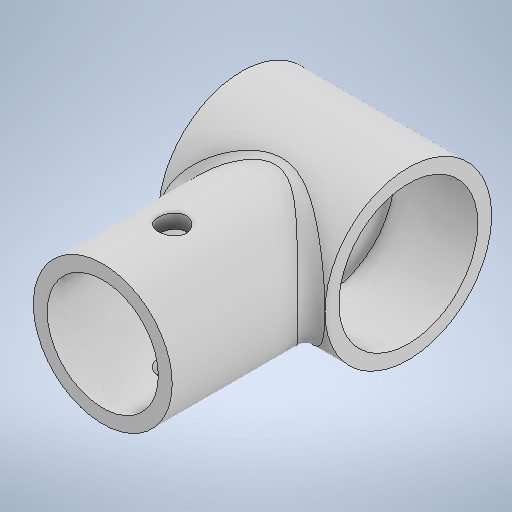
# Autodesk Inventor part: bielle rocker
Saved by Autodesk Inventor 2026.2 (Build 302298010, 298A)
## iProperties
Created: 2026-03-19
Part Number: bielle rocker
Material: Générique
Document SubType Name: Modeling
Designer: genon
Density: 1 g/cm^3
Appearance: Par défaut
Author: genon
Autodesk Inventor part; units mm, degrees
ref_plane "YZ Plane" through (0, 0, 0) normal (1, 0, 0) x (0, 1, 0)
ref_plane "XY Plane" through (0, 0, 0) normal (0, 0, 1) x (1, 0, 0)
sketch "Esquisse2" plane through (0, 0, 0) normal (0, 0, 1) x (1, 0, 0)
  circle A0 centre (0, 0) radius 4
  circle A1 centre (0, 0) radius 5
  dimension "d0" = 8
  dimension "d1" = 10
  constraints: 2 centre point, 2 coincident
  measures "d0" diameter of A0
  measures "d1" diameter of A1
extrude "Extrusion1" add sketch "Esquisse2" along normal blind 10
sketch "Esquisse3" plane through (0, 0, 0) normal (1, 0, 0) x (0, 1, 0)
  line L0 (0, 0) -> (0, -6)
  circle A0 centre (0, -6) radius 5
  circle A1 centre (0, -6) radius 6
  dimension "d4" = 6
  dimension "d5" = 10
  dimension "d6" = 12
  constraints: 2 centre point, 2 coincident, 2 end point, 1 vertical
  measures "d4" distance of L0.start L0.end
  measures "d5" diameter of A0
  measures "d6" diameter of A1
extrude "Extrusion2" add sketch "Esquisse3" along normal mid plane 12
sketch "Esquisse4" plane through (0, 0, 0) normal (1, 0, 0) x (0, 1, 0)
  circle A0 centre (0, -6) radius 5 projected
  line L0 (0, -11) -> (0, -1)
  circle A1 centre (0, -6) radius 2.75
  circle A2 centre (0, -6) radius 5
  line L1 (5, 0) -> (0, 0) projected
  line L2 (5, 0) -> (-5, 0)
  line L3 (-5, 0) -> (-5, -12)
  line L4 (-5, -12) -> (5, -12)
  line L5 (5, -12) -> (5, 0)
  point P0 (5, -6)
  point P1 (-5, -6)
  point P2 (-5, 0)
  dimension "d9" = 5.5
  dimension "d12" = 10
  dimension "d13" = 12
  constraints: 10 end point, 2 centre point, 2 coincident, 2 parallel, 2 point on circle, 1 concentric, 1 horizontal, 1 perpendicular, 1 vertical
  measures "d9" diameter of A1
  measures "d12" distance of L4.end L3.end
  measures "d13" distance of L3.end L2.end
extrude "Extrusion3" add sketch "Esquisse4" against normal blind 6 contours A0 L0 A1 | L0 A1 A0
sketch "Esquisse9" plane through (0, 0, 0) normal (0, 0, -1) x (-1, 0, 0)
  circle A0 centre (0, 0) radius 4 projected
  circle A1 centre (0, 0) radius 5 projected
extrude "Extrusion7" add sketch "Esquisse9" along normal blind 5
fillet "Congé6" radius 1 2 edges at (0.0212, -5, -2.6833) (0.0142, 5, -2.6833)
sketch "Esquisse10" plane through (6, 0, -6) normal (1, 0, 0) x (0, 0, -1)
  circle A0 centre (0, 0) radius 2.75 projected
  circle A1 centre (0, 0) radius 5 projected
  point P0 (-6, 0)
extrude "Extrusion8" cut sketch "Esquisse10" against normal up to surface (6 mm away)
sketch "Esquisse11" plane through (6, 0, -6) normal (1, 0, 0) x (0, 0, -1)
  circle A0 centre (0, 0) radius 2.75 projected
  point P0 (-6, 0)
extrude "Extrusion9" cut sketch "Esquisse11" against normal through all
sketch "Esquisse12" plane through (0, 0, 0) normal (0, 0, 1) x (1, 0, 0)
  spline S0 degree 6 poles (-4, 0) (-4, -0.1706) (-3.9913, -0.3409) (-3.9739, -0.5097) (-3.9481, -0.6758) (-3.9146, -0.8378) (-3.8162, -1.2211) (-3.7439, -1.4367) (-3.6595, -1.641) (-3.5648, -1.8337) (-3.4614, -2.0148) (-3.1972, -2.4201) (-3.0291, -2.6346) (-2.8495, -2.8288) (-2.6603, -3.0042) (-2.4625, -3.162) (-2.0833, -3.4211) (-1.9043, -3.5274) (-1.72, -3.6219) (-1.5309, -3.7046) (-1.3372, -3.7755) (-0.9557, -3.8889) (-0.7684, -3.933) (-0.5783, -3.9664) (-0.3864, -3.9888) (-0.1933, -4) (0.1946, -4) (0.3888, -3.9886) (0.582, -3.966) (0.7732, -3.9322) (0.9617, -3.8875) (1.3378, -3.775) (1.5253, -3.7064) (1.7085, -3.6267) (1.8872, -3.536) (2.0609, -3.4342) (2.3863, -3.2158) (2.5387, -3.1005) (2.6863, -2.9752) (2.8286, -2.8395) (2.965, -2.6927) (3.2054, -2.3992) (3.3113, -2.2554) (3.4117, -2.1027) (3.5058, -1.9409) (3.5927, -1.7696) (3.7304, -1.4514) (3.785, -1.3084) (3.8339, -1.1601) (3.8765, -1.0069) (3.9122, -0.8493) (3.9599, -0.576) (3.9758, -0.4626) (3.9879, -0.3478) (3.996, -0.2322) (4, -0.1161) (4, 0) knots 0 0 0 0 0 0 0 0.064971 0.064971 0.064971 0.064971 0.064971 0.158683 0.158683 0.158683 0.158683 0.158683 0.289146 0.289146 0.289146 0.289146 0.289146 0.398574 0.398574 0.398574 0.398574 0.398574 0.499968 0.499968 0.499968 0.499968 0.499968 0.60201 0.60201 0.60201 0.60201 0.60201 0.707934 0.707934 0.707934 0.707934 0.707934 0.80694 0.80694 0.80694 0.80694 0.80694 0.891528 0.891528 0.891528 0.891528 0.891528 0.955662 0.955662 0.955662 0.955662 0.955662 1 1 1 1 1 1 1 projected
  spline S1 degree 6 poles (4, 0) (4, 0.1704) (3.9913, 0.3407) (3.9739, 0.5098) (3.9481, 0.676) (3.9146, 0.8381) (3.8162, 1.2211) (3.7439, 1.4367) (3.6595, 1.641) (3.5648, 1.8337) (3.4614, 2.0148) (3.1948, 2.4239) (3.0236, 2.6415) (2.8408, 2.8382) (2.6481, 3.0155) (2.4465, 3.1747) (2.0632, 3.4332) (1.8841, 3.5382) (1.6998, 3.6314) (1.5107, 3.7129) (1.3171, 3.7826) (0.9387, 3.8928) (0.7546, 3.9354) (0.5679, 3.9676) (0.3794, 3.9892) (0.1898, 4) (-0.1287, 4) (-0.2573, 3.995) (-0.3856, 3.9851) (-0.5133, 3.9703) (-0.6401, 3.9505) (-0.83, 3.9135) (-0.8939, 3.8997) (-0.9576, 3.8847) (-1.0208, 3.8684) (-1.0837, 3.8509) (-1.3416, 3.7738) (-1.5327, 3.7036) (-1.7195, 3.6219) (-1.9015, 3.5287) (-2.0782, 3.424) (-2.4026, 3.2034) (-2.5514, 3.0898) (-2.6954, 2.9665) (-2.8344, 2.8332) (-2.9678, 2.6893) (-3.2054, 2.3992) (-3.3113, 2.2554) (-3.4117, 2.1027) (-3.5058, 1.9409) (-3.5927, 1.7696) (-3.771, 1.3574) (-3.8583, 1.108) (-3.9276, 0.8436) (-3.9756, 0.568) (-4, 0.2854) (-4, 0) knots 0 0 0 0 0 0 0 0.064926 0.064926 0.064926 0.064926 0.064926 0.158737 0.158737 0.158737 0.158737 0.158737 0.291447 0.291447 0.291447 0.291447 0.291447 0.400728 0.400728 0.400728 0.400728 0.400728 0.50039 0.50039 0.50039 0.50039 0.50039 0.567943 0.567943 0.567943 0.567943 0.567943 0.602493 0.602493 0.602493 0.602493 0.602493 0.710518 0.710518 0.710518 0.710518 0.710518 0.807398 0.807398 0.807398 0.807398 0.807398 0.891975 0.891975 0.891975 0.891975 0.891975 1 1 1 1 1 1 1 projected
  spline S2 degree 2 poles (5, 0) (5, 8.6603) (-2.5, 4.3301) (-10, 0) (-2.5, -4.3301) (5, -8.6603) (5, 0) knots 0 0 0 0.333333 0.333333 0.666667 0.666667 1 1 1 weights 1 0.5 1 0.5 1 0.5 1 projected
  point P0 (0, 0)
  constraints: 2 horizontal alignment, 1 other
extrude "Extrusion10" add sketch "Esquisse12" against normal blind 2 contours S1 S0 | S2
sketch "Esquisse13" plane through (6, 0, -6) normal (1, 0, 0) x (0, 0, -1)
  circle A0 centre (0, 0) radius 5 projected
  point P0 (-6, 0)
extrude "Extrusion11" cut sketch "Esquisse13" against normal up to surface (6 mm away)
ref_plane "Plan de construction2" through (0, 5.5, 0) normal (0, 1, 0) x (-1, 0, 0)
sketch "Esquisse14" plane through (0, 5.5, 0) normal (0, 1, 0) x (-1, 0, 0)
  line L0 (-4, 10) -> (4, 10) projected
  line L1 (0, 10) -> (0, 5)
  point P0 (0, 0)
  dimension "d51" = 5
  constraints: 2 end point, 1 coincident, 1 midpoint, 1 vertical
  measures "d51" distance of L1.start L1.end
hole "Perçage2" at (0, 5.5, 5) direction (0, -1, 0) diameter 2 end through all
